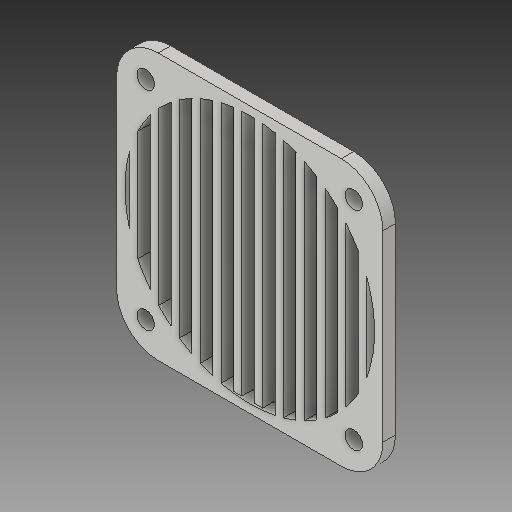
# Autodesk Inventor part: Fan_blend
Saved by Autodesk Inventor 2019.3 (Build 233278000, 278)
## iProperties
Created: 2020-10-09
Part Number: Fan_blend
Material: Generisch
Document SubType Name: Modeling
Designer: Nicolas Frick
Density: 1 g/cm^3
Appearance: Vorgabe
Author: Nicolas Frick
Autodesk Inventor part; units mm, degrees
ref_plane "YZ Plane" through (0, 0, 0) normal (1, 0, 0) x (0, 1, 0)
ref_plane "XZ Plane" through (0, 0, 0) normal (0, 1, 0) x (-1, 0, 0)
ref_plane "XY Plane" through (0, 0, 0) normal (0, 0, 1) x (1, 0, 0)
sketch "Skizze1" plane through (0, 0, 0) normal (0, 0, 1) x (1, 0, 0)
  line L0 (-41.5, 35.6804) -> (-41.5, -22.9) construction
  line L1 (-41.5, -22.9) -> (-43.9777, -22.9) construction
  line L2 (-43.9777, -22.9) -> (-43.9777, 35.6804) construction
  line L3 (-43.9777, 35.6804) -> (-41.5, 35.6804) construction
  line L4 (-47.5, 35.6804) -> (-47.5, -0.041) construction
  line L5 (-47.5, -0.041) -> (-49.9777, -0.041) construction
  line L6 (-49.9777, -0.041) -> (-49.9777, 35.6804) construction
  line L7 (-49.9777, 35.6804) -> (-47.5, 35.6804) construction
  circle A0 centre (-47.5, -3) radius 1.35 construction
  line L8 (36.5, 27.1) -> (36.5, -35.7623) construction
  line L9 (36.5, -35.7623) -> (34.0223, -35.7623) construction
  line L10 (34.0223, -35.7623) -> (34.0223, 27.1) construction
  line L11 (34.0223, 27.1) -> (36.5, 27.1) construction
  line L12 (30.5, -25.9706) -> (30.5, -35.7623) construction
  line L13 (30.5, -35.7623) -> (28.0223, -35.7623) construction
  line L14 (28.0223, -35.7623) -> (28.0223, -25.9706) construction
  line L15 (28.0223, -25.9706) -> (30.5, -25.9706) construction
  line L16 (18.5, -28.5) -> (18.5, -35.7623) construction
  line L17 (18.5, -35.7623) -> (16.0223, -35.7623) construction
  line L18 (16.0223, -35.7623) -> (16.0223, -28.5) construction
  line L19 (16.0223, -28.5) -> (18.5, -28.5) construction
  line L20 (-29.5, -16.7561) -> (-29.5, -22.9) construction
  line L21 (-29.5, -22.9) -> (-31.9777, -22.9) construction
  line L22 (-31.9777, -22.9) -> (-31.9777, -16.7561) construction
  line L23 (-31.9777, -16.7561) -> (-29.5, -16.7561) construction
  line L24 (-25.9777, 30.1243) -> (-25.9777, 35.6804) construction
  line L25 (-25.9777, 35.6804) -> (-23.5, 35.6804) construction
  line L26 (-23.5, 35.6804) -> (-23.5, 30.1243) construction
  line L27 (-23.5, 30.1243) -> (-25.9777, 30.1243) construction
  line L28 (16.0223, 31.6466) -> (16.0223, 35.6804) construction
  line L29 (16.0223, 35.6804) -> (18.5, 35.6804) construction
  line L30 (18.5, 35.6804) -> (18.5, 31.6466) construction
  line L31 (18.5, 31.6466) -> (16.0223, 31.6466) construction
  line L32 (-5.5, -32.1312) -> (-5.5, -35.7623) construction
  line L33 (-5.5, -35.7623) -> (-7.9777, -35.7623) construction
  line L34 (-7.9777, -35.7623) -> (-7.9777, -32.1312) construction
  line L35 (-7.9777, -32.1312) -> (-5.5, -32.1312) construction
  line L36 (10.0223, 32.8979) -> (10.0223, 35.6804) construction
  line L37 (10.0223, 35.6804) -> (12.5, 35.6804) construction
  line L38 (12.5, 35.6804) -> (12.5, 32.8979) construction
  line L39 (12.5, 32.8979) -> (10.0223, 32.8979) construction
  line L40 (-7.9777, 33.0955) -> (-7.9777, 35.6804) construction
  line L41 (-7.9777, 35.6804) -> (-5.5, 35.6804) construction
  line L42 (-5.5, 35.6804) -> (-5.5, 33.0955) construction
  line L43 (-5.5, 33.0955) -> (-7.9777, 33.0955) construction
  line L44 (0.5, -33.9467) -> (0.5, -35.7623) construction
  line L45 (0.5, -35.7623) -> (-1.9777, -35.7623) construction
  line L46 (-1.9777, -35.7623) -> (-1.9777, -33.9467) construction
  line L47 (-1.9777, -33.9467) -> (0.5, -33.9467) construction
  line L48 (-1.9777, 34.0902) -> (-1.9777, 35.6804) construction
  line L49 (-1.9777, 35.6804) -> (0.5, 35.6804) construction
  line L50 (0.5, 35.6804) -> (0.5, 34.0902) construction
  line L51 (0.5, 34.0902) -> (-1.9777, 34.0902) construction
  line L52 (6.5, -33.9467) -> (6.5, -35.7623) construction
  line L53 (6.5, -35.7623) -> (4.0223, -35.7623) construction
  line L54 (4.0223, -35.7623) -> (4.0223, -33.9467) construction
  line L55 (4.0223, -33.9467) -> (6.5, -33.9467) construction
  line L56 (4.0223, 32.8979) -> (4.0223, 35.6804) construction
  line L57 (4.0223, 35.6804) -> (6.5, 35.6804) construction
  line L58 (6.5, 35.6804) -> (6.5, 32.8979) construction
  line L59 (6.5, 32.8979) -> (4.0223, 32.8979) construction
  line L60 (-13.9777, 32.5) -> (-13.9777, 35.6804) construction
  line L61 (-13.9777, 35.6804) -> (-11.5, 35.6804) construction
  line L62 (-11.5, 35.6804) -> (-11.5, 32.5) construction
  line L63 (-11.5, 32.5) -> (-13.9777, 32.5) construction
  line L64 (12.5, -32.1312) -> (12.5, -35.7623) construction
  line L65 (12.5, -35.7623) -> (10.0223, -35.7623) construction
  line L66 (10.0223, -35.7623) -> (10.0223, -32.1312) construction
  line L67 (10.0223, -32.1312) -> (12.5, -32.1312) construction
  line L68 (-19.9777, 31.3064) -> (-19.9777, 35.6804) construction
  line L69 (-19.9777, 35.6804) -> (-17.5, 35.6804) construction
  line L70 (-17.5, 35.6804) -> (-17.5, 31.3064) construction
  line L71 (-17.5, 31.3064) -> (-19.9777, 31.3064) construction
  line L72 (22.0223, 30) -> (22.0223, 35.6804) construction
  line L73 (22.0223, 35.6804) -> (24.5, 35.6804) construction
  line L74 (24.5, 35.6804) -> (24.5, 30) construction
  line L75 (24.5, 30) -> (22.0223, 30) construction
  line L76 (-29.5, 27.1) -> (-29.5, 20.9081) construction
  line L77 (-29.5, 20.9081) -> (-31.9777, 20.9081) construction
  line L78 (-31.9777, 20.9081) -> (-31.9777, 27.1) construction
  line L79 (-31.9777, 27.1) -> (-29.5, 27.1) construction
  line L80 (24.5, -28.5) -> (24.5, -35.7623) construction
  line L81 (24.5, -35.7623) -> (22.0223, -35.7623) construction
  line L82 (22.0223, -35.7623) -> (22.0223, -28.5) construction
  line L83 (22.0223, -28.5) -> (24.5, -28.5) construction
  line L84 (-49.9777, -22.9) -> (-49.9777, -6.1402) construction
  line L85 (-49.9777, -6.1402) -> (-47.5, -6.1402) construction
  line L86 (-47.5, -6.1402) -> (-47.5, -22.9) construction
  line L87 (-47.5, -22.9) -> (-49.9777, -22.9) construction
  line L88 (46.0223, -27.1) -> (46.0223, 35.6804) construction
  line L89 (46.0223, 35.6804) -> (48.5, 35.6804) construction
  line L90 (48.5, 35.6804) -> (48.5, -27.1) construction
  line L91 (48.5, -27.1) -> (46.0223, -27.1) construction
  line L92 (40.0223, 35.6804) -> (42.5, 35.6804) construction
  line L93 (42.5, 35.6804) -> (42.5, -35.7623) construction
  line L94 (42.5, -35.7623) -> (40.0223, -35.7623) construction
  line L95 (40.0223, -35.7623) -> (40.0223, 35.6804) construction
  circle A1 centre (25, 25) radius 2.1 construction
  circle A2 centre (-25, 25) radius 2.1 construction
  circle A3 centre (-25, -25) radius 2.1 construction
  circle A4 centre (25, -25) radius 2.1 construction
  circle A5 centre (32, 32.5) radius 1.35 construction
  circle A6 centre (-30, 32.5) radius 1.35 construction
  circle A7 centre (47.5, -32.5) radius 1.35 construction
  line L96 (-35.5, 35.6804) -> (-35.5, -22.9) construction
  line L97 (-35.5, -22.9) -> (-37.9777, -22.9) construction
  line L98 (-37.9777, -22.9) -> (-37.9777, 35.6804) construction
  line L99 (-37.9777, 35.6804) -> (-35.5, 35.6804) construction
  line L100 (-52.5, -24.5) -> (-52.5, 37.5) construction
  line L101 (-52.5, -24.5) -> (-32.8176, -24.5) construction
  arc A8 (-32.8176, -24.5) -> (-11.4624, -29.9989) centre (-10.5668, 17.6958) ccw construction
  arc A9 (-9.5, -31.9985) -> (-11.4624, -29.9989) centre (-11.5, -31.9985) ccw construction
  line L102 (-9.5, -31.9985) -> (-9.5, -37.5) construction
  line L103 (52.5, -37.5) -> (-9.5, -37.5) construction
  line L104 (52.5, 37.5) -> (52.5, -37.5) construction
  line L105 (-52.5, 37.5) -> (52.5, 37.5) construction
  circle A10 centre (0, 0) radius 32 construction
  line L106 (-32, 32) -> (32, 32)
  line L107 (32, 32) -> (32, -32)
  line L108 (32, -32) -> (-32, -32)
  line L109 (-32, -32) -> (-32, 32)
  line L110 (-32, 32) -> (32, -32) construction
  line L111 (32, 32) -> (-32, -32) construction
  constraints: 12 end point, 2 midpoint, 2 parallel, 1 horizontal, 1 perpendicular
extrude "Extrusion1" add sketch "Skizze1" along normal blind 3
sketch "Skizze2" plane through (0, 0, 3) normal (0, 0, 1) x (1, 0, 0)
  circle A0 centre (0, 0) radius 30 projected
  circle A1 centre (25, 25) radius 2.1 projected
  circle A2 centre (-25, 25) radius 2.1 projected
  circle A3 centre (-25, -25) radius 2.1 projected
  circle A4 centre (25, -25) radius 2.1 projected
extrude "Extrusion2" cut sketch "Skizze2" against normal through all
sketch "Skizze3" plane through (0, 0, 3) normal (0, 0, 1) x (1, 0, 0)
  line L0 (28.0978, 30) -> (26.0978, 30)
  line L1 (26.0978, 30) -> (26.0978, -29.358)
  line L2 (26.0978, -29.358) -> (28.0978, -29.358)
  line L3 (28.0978, -29.358) -> (28.0978, 30)
  line L4 (32, 32) -> (-32, 32) construction
  line L5 (23.0978, 30) -> (21.0978, 30)
  line L6 (21.0978, 30) -> (21.0978, -29.358)
  line L7 (21.0978, -29.358) -> (23.0978, -29.358)
  line L8 (23.0978, -29.358) -> (23.0978, 30)
  line L9 (18.0978, 30) -> (16.0978, 30)
  line L10 (16.0978, 30) -> (16.0978, -29.358)
  line L11 (16.0978, -29.358) -> (18.0978, -29.358)
  line L12 (18.0978, -29.358) -> (18.0978, 30)
  line L13 (13.0978, 30) -> (11.0978, 30)
  line L14 (11.0978, 30) -> (11.0978, -29.358)
  line L15 (11.0978, -29.358) -> (13.0978, -29.358)
  line L16 (13.0978, -29.358) -> (13.0978, 30)
  line L17 (8.0978, 30) -> (6.0978, 30)
  line L18 (6.0978, 30) -> (6.0978, -29.358)
  line L19 (6.0978, -29.358) -> (8.0978, -29.358)
  line L20 (8.0978, -29.358) -> (8.0978, 30)
  line L21 (3.0978, 30) -> (1.0978, 30)
  line L22 (1.0978, 30) -> (1.0978, -29.358)
  line L23 (1.0978, -29.358) -> (3.0978, -29.358)
  line L24 (3.0978, -29.358) -> (3.0978, 30)
  line L25 (-1.9022, 30) -> (-3.9022, 30)
  line L26 (-3.9022, 30) -> (-3.9022, -29.358)
  line L27 (-3.9022, -29.358) -> (-1.9022, -29.358)
  line L28 (-1.9022, -29.358) -> (-1.9022, 30)
  line L29 (-6.9022, 30) -> (-8.9022, 30)
  line L30 (-8.9022, 30) -> (-8.9022, -29.358)
  line L31 (-8.9022, -29.358) -> (-6.9022, -29.358)
  line L32 (-6.9022, -29.358) -> (-6.9022, 30)
  line L33 (-11.9022, 30) -> (-13.9022, 30)
  line L34 (-13.9022, 30) -> (-13.9022, -29.358)
  line L35 (-13.9022, -29.358) -> (-11.9022, -29.358)
  line L36 (-11.9022, -29.358) -> (-11.9022, 30)
  line L37 (-16.9022, 30) -> (-18.9022, 30)
  line L38 (-18.9022, 30) -> (-18.9022, -29.358)
  line L39 (-18.9022, -29.358) -> (-16.9022, -29.358)
  line L40 (-16.9022, -29.358) -> (-16.9022, 30)
  line L41 (-21.9022, 30) -> (-23.9022, 30)
  line L42 (-23.9022, 30) -> (-23.9022, -29.358)
  line L43 (-23.9022, -29.358) -> (-21.9022, -29.358)
  line L44 (-21.9022, -29.358) -> (-21.9022, 30)
  line L45 (-26.9022, 30) -> (-28.9022, 30)
  line L46 (-28.9022, 30) -> (-28.9022, -29.358)
  line L47 (-28.9022, -29.358) -> (-26.9022, -29.358)
  line L48 (-26.9022, -29.358) -> (-26.9022, 30)
  point P0 (0, 0)
  dimension "d4" = 2
  dimension "d7" = 5
  constraints: 96 end point, 2 horizontal, 2 parallel, 1 perpendicular, 88 other
  measures "d4" distance of L2.end L1.end
  measures "d7" distance of L0.start L5.start
extrude "Extrusion3" add sketch "Skizze3" against normal blind 3
sketch "Skizze4" plane through (0, 0, 3) normal (0, 0, 1) x (1, 0, 0)
  arc A0 (-23.9022, 26.7902) -> (-26.9022, 25.8897) centre (-25, 25) ccw projected
  arc A1 (26.0978, 26.7902) -> (23.0978, 25.8897) centre (25, 25) ccw projected
  arc A2 (26.0978, -23.2098) -> (23.0978, -24.1103) centre (25, -25) ccw projected
  arc A3 (-23.9022, -23.2098) -> (-26.9022, -24.1103) centre (-25, -25) ccw projected
  circle A4 centre (-25, 25) radius 2.1
  circle A5 centre (25, 25) radius 2.1
  circle A6 centre (25, -25) radius 2.1
  circle A7 centre (-25, -25) radius 2.1
  point P0 (0, 0)
  constraints: 4 centre point, 4 coincident
extrude "Extrusion4" cut sketch "Skizze4" against normal blind 3
fillet "Rundung1" radius 10 4 edges at (32, 32, 1.5) (32, -32, 1.5) (-32, 32, 1.5) (-32, -32, 1.5)
